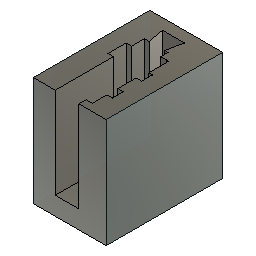
Endstop8 v4 (Autodesk Fusion 360 design; units mm, degrees)
Autodesk Fusion 360 part; units mm, degrees
note: some values were not read from the file. Chosen so that the rebuilt part matches the saved one: which face or edge a step refers to. Set by a fixed rule: which sketch regions a step uses.
(part 1 of 2)
sketch "Skizze1" plane through (0, 0, 0) normal (0, 0, 1) x (1, 0, 0)
  line L0 (0, 0) -> (20, 0)
  line L1 (20, 0) -> (20, -32)
  line L2 (20, -32) -> (0, -32)
  line L3 (0, -32) -> (0, 0)
  dimension "d1" = 20
  dimension "d2" = 32
  constraint horizontal L0
  constraint vertical L1
  constraint horizontal L2
  constraint vertical L3
  constraint coincident L0.start L3.end
  measures "d1" distance of L0.start L0.end
  measures "d2" distance of L0.start L2.end
extrude "Extrusion1" add sketch "Skizze1" along normal blind 25
sketch "Skizze2" plane through (0, 0, 25) normal (0, 0, 1) x (-1, 0, 0)
  line L0 (0, 32) -> (-20, 32)
  line L1 (-20, 32) -> (-20, 0)
  line L2 (-20, 0) -> (0, 0)
  line L3 (0, 0) -> (0, 32)
  line L4 (-12.516, 32) -> (-4.516, 32)
  line L5 (-4.516, 32) -> (-4.516, 10)
  line L6 (-4.516, 10) -> (-12.516, 10)
  line L7 (-12.516, 10) -> (-12.516, 32)
  dimension "d5" = 8
  dimension "d6" = 22
  constraint horizontal L4
  constraint vertical L5
  constraint horizontal L6
  constraint vertical L7
  constraint coincident L0 L4.start
  measures "d5" distance of L4.start L4.end
  measures "d6" distance of L4.start L6.end
extrude "Extrusion2" cut sketch "Skizze2" against normal blind 100 contours L0 L4 L5 L6 L7
sketch "Skizze3" plane through (0, 0, 25) normal (0, 0, 1) x (-1, 0, 0)
  line L0 (-12.516, 10) -> (-12.516, 32)
  line L1 (-12.516, 32) -> (-20, 32)
  line L2 (-20, 32) -> (-20, 0)
  line L3 (-20, 0) -> (0, 0)
  line L4 (0, 0) -> (0, 32)
  line L5 (0, 32) -> (-4.516, 32)
  line L6 (-4.516, 32) -> (-4.516, 10)
  line L7 (-4.516, 10) -> (-12.516, 10)
  line L8 (-12.516, 25.5233) -> (-14.516, 25.5233)
  line L9 (-14.516, 25.5233) -> (-14.516, 23.5233)
  line L10 (-14.516, 23.5233) -> (-12.516, 23.5233)
  line L11 (-12.516, 23.5233) -> (-12.516, 25.5233)
  dimension "d9" = 2
  dimension "d10" = 2
  constraint horizontal L8
  constraint vertical L9
  constraint horizontal L10
  constraint vertical L11
  constraint coincident L0 L8.start
  measures "d9" distance of L8.start L8.end
  measures "d10" distance of L8.start L10.end
extrude "Extrusion3" cut sketch "Skizze3" against normal blind 100 contours L0 L8 L9 L10 L11
sketch "Skizze4" plane through (0, 0, 25) normal (0, 0, 1) x (-1, 0, 0)
  line L0 (-14.516, 25.5233) -> (-12.516, 25.5233)
  line L1 (-12.516, 25.5233) -> (-12.516, 32)
  line L2 (-12.516, 32) -> (-20, 32)
  line L3 (-20, 32) -> (-20, 0)
  line L4 (-20, 0) -> (0, 0)
  line L5 (0, 0) -> (0, 32)
  line L6 (0, 32) -> (-4.516, 32)
  line L7 (-4.516, 32) -> (-4.516, 10)
  line L8 (-4.516, 10) -> (-12.516, 10)
  line L9 (-12.516, 10) -> (-12.516, 23.5233)
  line L10 (-12.516, 23.5233) -> (-14.516, 23.5233)
  line L11 (-14.516, 23.5233) -> (-14.516, 25.5233)
  line L12 (-12.516, 17.5114) -> (-14.516, 17.5114)
  line L13 (-14.516, 17.5114) -> (-14.516, 15.5114)
  line L14 (-14.516, 15.5114) -> (-12.516, 15.5114)
  line L15 (-12.516, 15.5114) -> (-12.516, 17.5114)
  dimension "d13" = 2
  dimension "d14" = 2
  constraint horizontal L12
  constraint vertical L13
  constraint horizontal L14
  constraint vertical L15
  constraint coincident L9 L12.start
  measures "d13" distance of L12.start L12.end
  measures "d14" distance of L12.start L14.end
extrude "Extrusion4" cut sketch "Skizze4" against normal blind 100 contours L9 L12 L13 L14 L15
sketch "Skizze5" plane through (0, 0, 25) normal (0, 0, 1) x (-1, 0, 0)
  line L0 (-12.516, 15.5114) -> (-14.516, 15.5114)
  line L1 (-14.516, 15.5114) -> (-14.516, 17.5114)
  line L2 (-14.516, 17.5114) -> (-12.516, 17.5114)
  line L3 (-12.516, 17.5114) -> (-12.516, 23.5233)
  line L4 (-12.516, 23.5233) -> (-14.516, 23.5233)
  line L5 (-14.516, 23.5233) -> (-14.516, 25.5233)
  line L6 (-14.516, 25.5233) -> (-12.516, 25.5233)
  line L7 (-12.516, 25.5233) -> (-12.516, 32)
  line L8 (-12.516, 32) -> (-20, 32)
  line L9 (-20, 32) -> (-20, 0)
  line L10 (-20, 0) -> (0, 0)
  line L11 (0, 0) -> (0, 32)
  line L12 (0, 32) -> (-4.516, 32)
  line L13 (-4.516, 32) -> (-4.516, 10)
  line L14 (-4.516, 10) -> (-12.516, 10)
  line L15 (-12.516, 10) -> (-12.516, 15.5114)
  line L16 (-12.516, 30.0118) -> (-14.216, 30.0118)
  line L17 (-14.216, 30.0118) -> (-14.216, 10.0118)
  line L18 (-14.216, 10.0118) -> (-12.516, 10.0118)
  line L19 (-12.516, 10.0118) -> (-12.516, 30.0118)
  dimension "d17" = 1.7
  dimension "d18" = 20
  constraint horizontal L16
  constraint vertical L17
  constraint horizontal L18
  constraint vertical L19
  constraint coincident L7 L16.start
  measures "d17" distance of L16.start L16.end
  measures "d18" distance of L16.start L18.end
extrude "Extrusion5" cut sketch "Skizze5" against normal blind 100 contours L0 L15 L17 L18 L19 | L2 L3 L4 L17 L19 | L6 L7 L16 L17 L19
sketch "Skizze6" plane through (0, 0, 25) normal (0, 0, 1) x (-1, 0, 0)
  line L0 (-12.516, 10.0118) -> (-14.216, 10.0118)
  line L1 (-14.216, 10.0118) -> (-14.216, 15.5114)
  line L2 (-14.216, 15.5114) -> (-14.516, 15.5114)
  line L3 (-14.516, 15.5114) -> (-14.516, 17.5114)
  line L4 (-14.516, 17.5114) -> (-14.216, 17.5114)
  line L5 (-14.216, 17.5114) -> (-14.216, 23.5233)
  line L6 (-14.216, 23.5233) -> (-14.516, 23.5233)
  line L7 (-14.516, 23.5233) -> (-14.516, 25.5233)
  line L8 (-14.516, 25.5233) -> (-14.216, 25.5233)
  line L9 (-14.216, 25.5233) -> (-14.216, 30.0118)
  line L10 (-14.216, 30.0118) -> (-12.516, 30.0118)
  line L11 (-12.516, 30.0118) -> (-12.516, 32)
  line L12 (-12.516, 32) -> (-20, 32)
  line L13 (-20, 32) -> (-20, 0)
  line L14 (-20, 0) -> (0, 0)
  line L15 (0, 0) -> (0, 32)
  line L16 (0, 32) -> (-4.516, 32)
  line L17 (-4.516, 32) -> (-4.516, 10)
  line L18 (-4.516, 10) -> (-12.516, 10)
  line L19 (-12.516, 10) -> (-12.516, 10.0118)
  line L20 (-14.516, 23.5233) -> (-15.716, 23.5233)
  line L21 (-15.716, 23.5233) -> (-15.716, 25.5)
  line L22 (-15.716, 25.5) -> (-14.516, 25.5)
  line L23 (-14.516, 25.5) -> (-14.516, 23.5233)
  dimension "d21" = 1.2
  constraint horizontal L20
  constraint vertical L21
  constraint horizontal L22
  constraint vertical L23
  constraint coincident L6.end L7.start
  measures "d21" distance of L6.end L20.end
extrude "Extrusion6" cut sketch "Skizze6" against normal blind 100 contours L7 L20 L21 L22 L23
sketch "Skizze7" plane through (0, 0, 25) normal (0, 0, 1) x (-1, 0, 0)
  line L0 (-14.216, 23.5233) -> (-15.716, 23.5233)
  line L1 (-15.716, 23.5233) -> (-15.716, 25.5)
  line L2 (-15.716, 25.5) -> (-14.516, 25.5)
  line L3 (-14.516, 25.5) -> (-14.516, 25.5233)
  line L4 (-14.516, 25.5233) -> (-14.216, 25.5233)
  line L5 (-14.216, 25.5233) -> (-14.216, 30.0118)
  line L6 (-14.216, 30.0118) -> (-12.516, 30.0118)
  line L7 (-12.516, 30.0118) -> (-12.516, 32)
  line L8 (-12.516, 32) -> (-20, 32)
  line L9 (-20, 32) -> (-20, 0)
  line L10 (-20, 0) -> (0, 0)
  line L11 (0, 0) -> (0, 32)
  line L12 (0, 32) -> (-4.516, 32)
  line L13 (-4.516, 32) -> (-4.516, 10)
  line L14 (-4.516, 10) -> (-12.516, 10)
  line L15 (-12.516, 10) -> (-12.516, 10.0118)
  line L16 (-12.516, 10.0118) -> (-14.216, 10.0118)
  line L17 (-14.216, 10.0118) -> (-14.216, 15.5114)
  line L18 (-14.216, 15.5114) -> (-14.516, 15.5114)
  line L19 (-14.516, 15.5114) -> (-14.516, 17.5114)
  line L20 (-14.516, 17.5114) -> (-14.216, 17.5114)
  line L21 (-14.216, 17.5114) -> (-14.216, 23.5233)
  line L22 (-14.516, 17.5114) -> (-15.716, 17.5114)
  line L23 (-15.716, 17.5114) -> (-15.716, 15.5)
  line L24 (-15.716, 15.5) -> (-14.516, 15.5)
  line L25 (-14.516, 15.5) -> (-14.516, 17.5114)
  dimension "d24" = 1.2
  constraint horizontal L22
  constraint vertical L23
  constraint horizontal L24
  constraint vertical L25
  constraint coincident L19.end L20.start
  measures "d24" distance of L19.end L22.end
extrude "Extrusion7" cut sketch "Skizze7" against normal blind 100 contours L19 L22 L23 L24 L25
sketch "Skizze8" plane through (0, 0, 25) normal (0, 0, 1) x (-1, 0, 0)
  line L0 (-14.516, 15.5114) -> (-14.516, 15.5)
  line L1 (-14.516, 15.5) -> (-15.716, 15.5)
  line L2 (-15.716, 15.5) -> (-15.716, 17.5114)
  line L3 (-15.716, 17.5114) -> (-14.216, 17.5114)
  line L4 (-14.216, 17.5114) -> (-14.216, 23.5233)
  line L5 (-14.216, 23.5233) -> (-15.716, 23.5233)
  line L6 (-15.716, 23.5233) -> (-15.716, 25.5)
  line L7 (-15.716, 25.5) -> (-14.516, 25.5)
  line L8 (-14.516, 25.5) -> (-14.516, 25.5233)
  line L9 (-14.516, 25.5233) -> (-14.216, 25.5233)
  line L10 (-14.216, 25.5233) -> (-14.216, 30.0118)
  line L11 (-14.216, 30.0118) -> (-12.516, 30.0118)
  line L12 (-12.516, 30.0118) -> (-12.516, 32)
  line L13 (-12.516, 32) -> (-20, 32)
  line L14 (-20, 32) -> (-20, 0)
  line L15 (-20, 0) -> (0, 0)
  line L16 (0, 0) -> (0, 32)
  line L17 (0, 32) -> (-4.516, 32)
  line L18 (-4.516, 32) -> (-4.516, 10)
  line L19 (-4.516, 10) -> (-12.516, 10)
  line L20 (-12.516, 10) -> (-12.516, 10.0118)
  line L21 (-12.516, 10.0118) -> (-14.216, 10.0118)
  line L22 (-14.216, 10.0118) -> (-14.216, 15.5114)
  line L23 (-14.216, 15.5114) -> (-14.516, 15.5114)
  line L24 (-12.516, 10) -> (-4.516, 10)
  line L25 (-4.516, 10) -> (-4.516, 8)
  line L26 (-4.516, 8) -> (-12.516, 8)
  line L27 (-12.516, 8) -> (-12.516, 10)
  dimension "d27" = 8
  dimension "d28" = 2
  constraint horizontal L24
  constraint vertical L25
  constraint horizontal L26
  constraint vertical L27
  constraint coincident L19.end L20.start
  measures "d27" distance of L19.end L18.end
  measures "d28" distance of L19.end L26.end
extrude "Extrusion8" cut sketch "Skizze8" against normal blind 100 contours L19 L24 L25 L26 L27
hole "Bohrung1" at (8.516, -8, 25) direction (0, 0, -1) diameter 8 depth 1000 tip angle 180
sketch "Skizze12" plane through (0, 0, 25) normal (0, 0, 1) x (-1, 0, 0)
  arc A0 (-12.516, 8) -> (-4.516, 8) centre (-8.516, 8) ccw
  line L0 (-12.516, 8) -> (-12.516, 10.0118)
  line L1 (-12.516, 10.0118) -> (-14.216, 10.0118)
  line L2 (-14.216, 10.0118) -> (-14.216, 15.5114)
  line L3 (-14.216, 15.5114) -> (-14.516, 15.5114)
  line L4 (-14.516, 15.5114) -> (-14.516, 15.5)
  line L5 (-14.516, 15.5) -> (-15.716, 15.5)
  line L6 (-15.716, 15.5) -> (-15.716, 17.5114)
  line L7 (-15.716, 17.5114) -> (-14.216, 17.5114)
  line L8 (-14.216, 17.5114) -> (-14.216, 23.5233)
  line L9 (-14.216, 23.5233) -> (-15.716, 23.5233)
  line L10 (-15.716, 23.5233) -> (-15.716, 25.5)
  line L11 (-15.716, 25.5) -> (-14.516, 25.5)
  line L12 (-14.516, 25.5) -> (-14.516, 25.5233)
  line L13 (-14.516, 25.5233) -> (-14.216, 25.5233)
  line L14 (-14.216, 25.5233) -> (-14.216, 30.0118)
  line L15 (-14.216, 30.0118) -> (-12.516, 30.0118)
  line L16 (-12.516, 30.0118) -> (-12.516, 32)
  line L17 (-12.516, 32) -> (-20, 32)
  line L18 (-20, 32) -> (-20, 0)
  line L19 (-20, 0) -> (0, 0)
  line L20 (0, 0) -> (0, 32)
  line L21 (0, 32) -> (-4.516, 32)
  line L22 (-4.516, 32) -> (-4.516, 8)
  line L23 (-12.516, 10.0118) -> (-14.216, 10.0118)
  line L24 (-14.216, 10.0118) -> (-14.216, 9.5118)
  line L25 (-14.216, 9.5118) -> (-12.516, 9.5118)
  line L26 (-12.516, 9.5118) -> (-12.516, 10.0118)
  line L27 (-14.216, 14.9916) -> (-15.716, 14.9916)
  line L28 (-15.716, 14.9916) -> (-15.716, 17.9916)
  line L29 (-15.716, 17.9916) -> (-14.216, 17.9916)
  line L30 (-14.216, 17.9916) -> (-14.216, 14.9916)
  line L31 (-14.216, 23.0062) -> (-15.716, 23.0062)
  line L32 (-15.716, 23.0062) -> (-15.716, 26.0062)
  line L33 (-15.716, 26.0062) -> (-14.216, 26.0062)
  line L34 (-14.216, 26.0062) -> (-14.216, 23.0062)
  dimension "d47" = 1.7
  dimension "d48" = 0.5
  dimension "d49" = 1.5
  dimension "d50" = 3
  dimension "d51" = 1.5
  dimension "d52" = 3
  constraint horizontal L23
  constraint vertical L24
  constraint horizontal L25
  constraint vertical L26
  constraint coincident L0.end L1.start
  constraint horizontal L27
  constraint vertical L28
  constraint horizontal L29
  constraint vertical L30
  constraint coincident L2 L27.start
  constraint horizontal L31
  constraint vertical L32
  constraint horizontal L33
  constraint vertical L34
  constraint coincident L8 L31.start
  measures "d47" distance of L0.end L1.end
  measures "d48" distance of L0.end L25.end
  measures "d49" distance of L27.start L27.end
  measures "d50" distance of L27.start L29.end
  measures "d51" distance of L31.start L31.end
  measures "d52" distance of L31.start L33.end
extrude "Extrusion12" cut sketch "Skizze12" against normal blind 100 contours L0 L1 L23 L24 L25 L26 | L2 L3 L4 L5 L27 L28 L30 | L7 L8 L28 L29 L30 | L8 L9 L31 L32 L34 | L11 L12 L13 L14 L32 L33 L34
sketch "Skizze13" plane through (0, 0, 25) normal (0, 0, 1) x (-1, 0, 0)
  line L0 (-15.716, 14.9916) -> (-15.716, 17.9916)
  line L1 (-15.716, 17.9916) -> (-14.216, 17.9916)
  line L2 (-14.216, 17.9916) -> (-14.216, 23.0062)
  line L3 (-14.216, 23.0062) -> (-15.716, 23.0062)
  line L4 (-15.716, 23.0062) -> (-15.716, 26.0062)
  line L5 (-15.716, 26.0062) -> (-14.216, 26.0062)
  line L6 (-14.216, 26.0062) -> (-14.216, 30.0118)
  line L7 (-14.216, 30.0118) -> (-12.516, 30.0118)
  line L8 (-12.516, 30.0118) -> (-12.516, 32)
  line L9 (-12.516, 32) -> (-20, 32)
  line L10 (-20, 32) -> (-20, 0)
  line L11 (-20, 0) -> (0, 0)
  line L12 (0, 0) -> (0, 32)
  line L13 (0, 32) -> (-4.516, 32)
  line L14 (-4.516, 32) -> (-4.516, 8)
  arc A0 (-12.516, 8) -> (-4.516, 8) centre (-8.516, 8) ccw
  line L15 (-12.516, 8) -> (-12.516, 9.5118)
  line L16 (-12.516, 9.5118) -> (-14.216, 9.5118)
  line L17 (-14.216, 9.5118) -> (-14.216, 14.9916)
  line L18 (-14.216, 14.9916) -> (-15.716, 14.9916)
  line L19 (-12.516, 8) -> (-10, 8)
  line L20 (-10, 8) -> (-10, 4.2855)
  constraint coincident A0.start L15.start
  constraint perpendicular L15 L19
  constraint coincident A0 L20.end
  constraint perpendicular L19 L20
extrude "Extrusion13" add sketch "Skizze13" against normal blind 25 contours A0 L19 L20
sketch "Skizze14" plane through (0, 0, 25) normal (0, 0, 1) x (-1, 0, 0)
  line L0 (-15.716, 14.9916) -> (-15.716, 17.9916)
  line L1 (-15.716, 17.9916) -> (-14.216, 17.9916)
  line L2 (-14.216, 17.9916) -> (-14.216, 23.0062)
  line L3 (-14.216, 23.0062) -> (-15.716, 23.0062)
  line L4 (-15.716, 23.0062) -> (-15.716, 26.0062)
  line L5 (-15.716, 26.0062) -> (-14.216, 26.0062)
  line L6 (-14.216, 26.0062) -> (-14.216, 30.0118)
  line L7 (-14.216, 30.0118) -> (-12.516, 30.0118)
  line L8 (-12.516, 30.0118) -> (-12.516, 32)
  line L9 (-12.516, 32) -> (-20, 32)
  line L10 (-20, 32) -> (-20, 0)
  line L11 (-20, 0) -> (0, 0)
  line L12 (0, 0) -> (0, 32)
  line L13 (0, 32) -> (-4.516, 32)
  line L14 (-4.516, 32) -> (-4.516, 8)
  arc A0 (-10, 4.2855) -> (-4.516, 8) centre (-8.516, 8) ccw
  line L15 (-10, 4.2855) -> (-10, 8)
  line L16 (-10, 8) -> (-12.516, 8)
  line L17 (-12.516, 8) -> (-12.516, 9.5118)
  line L18 (-12.516, 9.5118) -> (-14.216, 9.5118)
  line L19 (-14.216, 9.5118) -> (-14.216, 14.9916)
  line L20 (-14.216, 14.9916) -> (-15.716, 14.9916)
  line L21 (-7.0738, 4.269) -> (-7.0738, 8)
  line L22 (-7.0738, 8) -> (-4.516, 8)
  constraint coincident A0 L21.start
  constraint parallel L12 L21
  constraint coincident L14.end A0.end
extrude "Extrusion14" add sketch "Skizze14" against normal blind 25 contours A0 L21 L22
sketch "Skizze15" plane through (0, 0, 25) normal (0, 0, 1) x (-1, 0, 0)
  line L0 (-15.716, 14.9916) -> (-15.716, 17.9916)
  line L1 (-15.716, 17.9916) -> (-14.216, 17.9916)
  line L2 (-14.216, 17.9916) -> (-14.216, 23.0062)
  line L3 (-14.216, 23.0062) -> (-15.716, 23.0062)
  line L4 (-15.716, 23.0062) -> (-15.716, 26.0062)
  line L5 (-15.716, 26.0062) -> (-14.216, 26.0062)
  line L6 (-14.216, 26.0062) -> (-14.216, 30.0118)
  line L7 (-14.216, 30.0118) -> (-12.516, 30.0118)
  line L8 (-12.516, 30.0118) -> (-12.516, 32)
  line L9 (-12.516, 32) -> (-20, 32)
  line L10 (-20, 32) -> (-20, 0)
  line L11 (-20, 0) -> (0, 0)
  line L12 (0, 0) -> (0, 32)
  line L13 (0, 32) -> (-4.516, 32)
  line L14 (-4.516, 32) -> (-4.516, 8)
  line L15 (-4.516, 8) -> (-7.0738, 8)
  line L16 (-7.0738, 8) -> (-7.0738, 4.269)
  arc A0 (-10, 4.2855) -> (-7.0738, 4.269) centre (-8.516, 8) ccw
  line L17 (-10, 4.2855) -> (-10, 8)
  line L18 (-10, 8) -> (-12.516, 8)
  line L19 (-12.516, 8) -> (-12.516, 9.5118)
  line L20 (-12.516, 9.5118) -> (-14.216, 9.5118)
  line L21 (-14.216, 9.5118) -> (-14.216, 14.9916)
  line L22 (-14.216, 14.9916) -> (-15.716, 14.9916)
  line L23 (-7.0738, 8) -> (-6.6738, 8)
  line L24 (-6.6738, 8) -> (-6.6738, 4.0061)
  line L25 (-6.6738, 4.0061) -> (-7.0738, 4.0061)
  line L26 (-7.0738, 4.0061) -> (-7.0738, 8)
  line L27 (-10, 8) -> (-10.4, 8)
  line L28 (-10.4, 8) -> (-10.4, 4.0061)
  line L29 (-10.4, 4.0061) -> (-10, 4.0061)
  line L30 (-10, 4.0061) -> (-10, 8)
  line L31 (-6.6738, 4.0061) -> (-10.4, 4.0061)
  line L32 (-10.4, 4.0061) -> (-10.4, 4.5457)
  line L33 (-10.4, 4.5457) -> (-6.6738, 4.5457)
  line L34 (-6.6738, 4.5457) -> (-6.6738, 4.0061)
  dimension "d59" = 0.4
  dimension "d60" = 0.4
  constraint horizontal L23
  constraint vertical L24
  constraint horizontal L25
  constraint vertical L26
  constraint coincident L15.end L16.start
  constraint horizontal L27
  constraint vertical L28
  constraint horizontal L29
  constraint vertical L30
  constraint coincident L17.end L18.start
  constraint horizontal L31
  constraint vertical L32
  constraint horizontal L33
  constraint vertical L34
  constraint coincident L28 L32.end
  measures "d59" distance of L15.end L23.end
  measures "d60" distance of L17.end L27.end
extrude "Extrusion15" cut sketch "Skizze15" against normal blind 30 contours L17 L18 L27 L28 L30 L33 | L17 L28 L29 L30 L31 L32 L33 | A0 L30 L31 | L16 L24 L25 L26 L31 L33 L34 | L15 L16 L23 L24 L26 L33 | A0 L26 L31
sketch "Skizze16" plane through (0, 0, 25) normal (0, 0, 1) x (-1, 0, 0)
  line L0 (-6.6738, 8) -> (-6.6738, 4.0061)
  line L1 (-6.6738, 4.0061) -> (-8.2952, 4.0061)
  arc A0 (-8.7369, 4.0061) -> (-8.2952, 4.0061) centre (-8.516, 8) ccw
  line L2 (-8.7369, 4.0061) -> (-10.4, 4.0061)
  line L3 (-10.4, 4.0061) -> (-10.4, 8)
  line L4 (-10.4, 8) -> (-12.516, 8)
  line L5 (-12.516, 8) -> (-12.516, 9.5118)
  line L6 (-12.516, 9.5118) -> (-14.216, 9.5118)
  line L7 (-14.216, 9.5118) -> (-14.216, 14.9916)
  line L8 (-14.216, 14.9916) -> (-15.716, 14.9916)
  line L9 (-15.716, 14.9916) -> (-15.716, 17.9916)
  line L10 (-15.716, 17.9916) -> (-14.216, 17.9916)
  line L11 (-14.216, 17.9916) -> (-14.216, 23.0062)
  line L12 (-14.216, 23.0062) -> (-15.716, 23.0062)
  line L13 (-15.716, 23.0062) -> (-15.716, 26.0062)
  line L14 (-15.716, 26.0062) -> (-14.216, 26.0062)
  line L15 (-14.216, 26.0062) -> (-14.216, 30.0118)
  line L16 (-14.216, 30.0118) -> (-12.516, 30.0118)
  line L17 (-12.516, 30.0118) -> (-12.516, 32)
  line L18 (-12.516, 32) -> (-20, 32)
  line L19 (-20, 32) -> (-20, 0)
  line L20 (-20, 0) -> (0, 0)
  line L21 (0, 0) -> (0, 32)
  line L22 (0, 32) -> (-4.516, 32)
  line L23 (-4.516, 32) -> (-4.516, 8)
  line L24 (-4.516, 8) -> (-6.6738, 8)
  line L25 (-4.516, 32) -> (-6.016, 32)
  line L26 (-6.016, 32) -> (-6.016, 8)
  line L27 (-6.016, 8) -> (-4.516, 8)
  line L28 (-4.516, 8) -> (-4.516, 32)
  dimension "d63" = 1.5
  constraint horizontal L25
  constraint vertical L26
  constraint horizontal L27
  constraint vertical L28
  constraint coincident L22.end L23.start
  measures "d63" distance of L22.end L25.end
extrude "Extrusion16" add sketch "Skizze16" against normal blind 25 contours L23 L24 L25 L26 L27 L28
sketch "Skizze17" plane through (0, 0, 25) normal (0, 0, 1) x (-1, 0, 0)
  line L0 (-6.6738, 8) -> (-6.6738, 4.0061)
  line L1 (-6.6738, 4.0061) -> (-8.2952, 4.0061)
  arc A0 (-8.7369, 4.0061) -> (-8.2952, 4.0061) centre (-8.516, 8) ccw
  line L2 (-8.7369, 4.0061) -> (-10.4, 4.0061)
  line L3 (-10.4, 4.0061) -> (-10.4, 8)
  line L4 (-10.4, 8) -> (-12.516, 8)
  line L5 (-12.516, 8) -> (-12.516, 9.5118)
  line L6 (-12.516, 9.5118) -> (-14.216, 9.5118)
  line L7 (-14.216, 9.5118) -> (-14.216, 14.9916)
  line L8 (-14.216, 14.9916) -> (-15.716, 14.9916)
  line L9 (-15.716, 14.9916) -> (-15.716, 17.9916)
  line L10 (-15.716, 17.9916) -> (-14.216, 17.9916)
  line L11 (-14.216, 17.9916) -> (-14.216, 23.0062)
  line L12 (-14.216, 23.0062) -> (-15.716, 23.0062)
  line L13 (-15.716, 23.0062) -> (-15.716, 26.0062)
  line L14 (-15.716, 26.0062) -> (-14.216, 26.0062)
  line L15 (-14.216, 26.0062) -> (-14.216, 30.0118)
  line L16 (-14.216, 30.0118) -> (-12.516, 30.0118)
  line L17 (-12.516, 30.0118) -> (-12.516, 32)
  line L18 (-12.516, 32) -> (-20, 32)
  line L19 (-20, 32) -> (-20, 0)
  line L20 (-20, 0) -> (0, 0)
  line L21 (0, 0) -> (0, 32)
  line L22 (0, 32) -> (-6.016, 32)
  line L23 (-6.016, 32) -> (-6.016, 8)
  line L24 (-6.016, 8) -> (-6.6738, 8)
  line L25 (-14.216, 14.9916) -> (-14.716, 14.9916)
  line L26 (-14.716, 14.9916) -> (-14.716, 9.513)
  line L27 (-14.716, 9.513) -> (-14.216, 9.513)
  line L28 (-14.216, 9.513) -> (-14.216, 14.9916)
  dimension "d66" = 0.5
  constraint horizontal L25
  constraint vertical L26
  constraint horizontal L27
  constraint vertical L28
  constraint coincident L7.end L8.start
  measures "d66" distance of L7.end L25.end
extrude "Extrusion17" cut sketch "Skizze17" against normal blind 25 contours L7 L8 L25 L26 L27 L28
sketch "Skizze18" plane through (0, 0, 25) normal (0, 0, 1) x (-1, 0, 0)
  line L0 (-14.216, 9.513) -> (-14.716, 9.513)
  line L1 (-14.716, 9.513) -> (-14.716, 14.9916)
  line L2 (-14.716, 14.9916) -> (-15.716, 14.9916)
  line L3 (-15.716, 14.9916) -> (-15.716, 17.9916)
  line L4 (-15.716, 17.9916) -> (-14.216, 17.9916)
  line L5 (-14.216, 17.9916) -> (-14.216, 23.0062)
  line L6 (-14.216, 23.0062) -> (-15.716, 23.0062)
  line L7 (-15.716, 23.0062) -> (-15.716, 26.0062)
  line L8 (-15.716, 26.0062) -> (-14.216, 26.0062)
  line L9 (-14.216, 26.0062) -> (-14.216, 30.0118)
  line L10 (-14.216, 30.0118) -> (-12.516, 30.0118)
  line L11 (-12.516, 30.0118) -> (-12.516, 32)
  line L12 (-12.516, 32) -> (-20, 32)
  line L13 (-20, 32) -> (-20, 0)
  line L14 (-20, 0) -> (0, 0)
  line L15 (0, 0) -> (0, 32)
  line L16 (0, 32) -> (-6.016, 32)
  line L17 (-6.016, 32) -> (-6.016, 8)
  line L18 (-6.016, 8) -> (-6.6738, 8)
  line L19 (-6.6738, 8) -> (-6.6738, 4.0061)
  line L20 (-6.6738, 4.0061) -> (-8.2952, 4.0061)
  arc A0 (-8.7369, 4.0061) -> (-8.2952, 4.0061) centre (-8.516, 8) ccw
  line L21 (-8.7369, 4.0061) -> (-10.4, 4.0061)
  line L22 (-10.4, 4.0061) -> (-10.4, 8)
  line L23 (-10.4, 8) -> (-12.516, 8)
  line L24 (-12.516, 8) -> (-12.516, 9.5118)
  line L25 (-12.516, 9.5118) -> (-14.216, 9.5118)
  line L26 (-14.216, 9.5118) -> (-14.216, 9.513)
  line L27 (-10.4, 8) -> (-11.4, 8)
  line L28 (-11.4, 8) -> (-11.4, 4.0168)
  line L29 (-11.4, 4.0168) -> (-10.4, 4.0168)
  line L30 (-10.4, 4.0168) -> (-10.4, 8)
  line L31 (-10.4, 8) -> (-11.6, 8)
  line L32 (-11.6, 8) -> (-11.6, 4.008)
  line L33 (-11.6, 4.008) -> (-10.4, 4.008)
  line L34 (-10.4, 4.008) -> (-10.4, 8)
  point P0 (-10.4, 4.0061)
  point P1 (-10.4, 8)
  point P2 (-10.4, 4.0061)
  dimension "d69" = 1
  dimension "d70" = 1.2
  constraint horizontal L27
  constraint vertical L28
  constraint horizontal L29
  constraint vertical L30
  constraint horizontal L31
  constraint vertical L32
  constraint horizontal L33
  constraint vertical L34
  measures "d69" distance of P1 L27.end
  measures "d70" distance of P1 L31.end
extrude "Extrusion18" cut sketch "Skizze18" against normal blind 30 contours L22 L23 L28 L29 L31 L32 L33 L34 | L22 L23 L27 L28 L29 L30 L31 L34
sketch "Skizze19" plane through (0, 0, 25) normal (0, 0, 1) x (-1, 0, 0)
  line L0 (-10.4, 4.008) -> (-11.6, 4.008)
  line L1 (-11.6, 4.008) -> (-11.6, 8)
  line L2 (-11.6, 8) -> (-12.516, 8)
  line L3 (-12.516, 8) -> (-12.516, 9.5118)
  line L4 (-12.516, 9.5118) -> (-14.216, 9.5118)
  line L5 (-14.216, 9.5118) -> (-14.216, 9.513)
  line L6 (-14.216, 9.513) -> (-14.716, 9.513)
  line L7 (-14.716, 9.513) -> (-14.716, 14.9916)
  line L8 (-14.716, 14.9916) -> (-15.716, 14.9916)
  line L9 (-15.716, 14.9916) -> (-15.716, 17.9916)
  line L10 (-15.716, 17.9916) -> (-14.216, 17.9916)
  line L11 (-14.216, 17.9916) -> (-14.216, 23.0062)
  line L12 (-14.216, 23.0062) -> (-15.716, 23.0062)
  line L13 (-15.716, 23.0062) -> (-15.716, 26.0062)
  line L14 (-15.716, 26.0062) -> (-14.216, 26.0062)
  line L15 (-14.216, 26.0062) -> (-14.216, 30.0118)
  line L16 (-14.216, 30.0118) -> (-12.516, 30.0118)
  line L17 (-12.516, 30.0118) -> (-12.516, 32)
  line L18 (-12.516, 32) -> (-20, 32)
  line L19 (-20, 32) -> (-20, 0)
  line L20 (-20, 0) -> (0, 0)
  line L21 (0, 0) -> (0, 32)
  line L22 (0, 32) -> (-6.016, 32)
  line L23 (-6.016, 32) -> (-6.016, 8)
  line L24 (-6.016, 8) -> (-6.6738, 8)
  line L25 (-6.6738, 8) -> (-6.6738, 4.0061)
  line L26 (-6.6738, 4.0061) -> (-8.2952, 4.0061)
  arc A0 (-8.7369, 4.0061) -> (-8.2952, 4.0061) centre (-8.516, 8) ccw
  line L27 (-8.7369, 4.0061) -> (-10.4, 4.0061)
  line L28 (-10.4, 4.0061) -> (-10.4, 4.008)
  line L29 (-6.016, 8) -> (-12.5254, 8)
  line L30 (-12.5254, 8) -> (-12.5254, 7.5)
  line L31 (-12.5254, 7.5) -> (-6.016, 7.5)
  line L32 (-6.016, 7.5) -> (-6.016, 8)
  dimension "d73" = 0.5
  constraint horizontal L29
  constraint vertical L30
  constraint horizontal L31
  constraint vertical L32
  constraint coincident L23.end L24.start
  measures "d73" distance of L23.end L31.end
extrude "Extrusion19" cut sketch "Skizze19" against normal blind 30 contours L1 L2 L29 L30 L31 | L24 L25 L29 L31 L32
sketch "Skizze20" plane through (0, 0, 25) normal (0, 0, 1) x (-1, 0, 0)
  line L0 (-6.016, 7.5) -> (-6.6738, 7.5)
  line L1 (-6.6738, 7.5) -> (-6.6738, 4.0061)
  line L2 (-6.6738, 4.0061) -> (-8.2952, 4.0061)
  arc A0 (-8.7369, 4.0061) -> (-8.2952, 4.0061) centre (-8.516, 8) ccw
  line L3 (-8.7369, 4.0061) -> (-10.4, 4.0061)
  line L4 (-10.4, 4.0061) -> (-10.4, 4.008)
  line L5 (-10.4, 4.008) -> (-11.6, 4.008)
  line L6 (-11.6, 4.008) -> (-11.6, 7.5)
  line L7 (-11.6, 7.5) -> (-12.5254, 7.5)
  line L8 (-12.5254, 7.5) -> (-12.5254, 8)
  line L9 (-12.5254, 8) -> (-12.516, 8)
  line L10 (-12.516, 8) -> (-12.516, 9.5118)
  line L11 (-12.516, 9.5118) -> (-14.216, 9.5118)
  line L12 (-14.216, 9.5118) -> (-14.216, 9.513)
  line L13 (-14.216, 9.513) -> (-14.716, 9.513)
  line L14 (-14.716, 9.513) -> (-14.716, 14.9916)
  line L15 (-14.716, 14.9916) -> (-15.716, 14.9916)
  line L16 (-15.716, 14.9916) -> (-15.716, 17.9916)
  line L17 (-15.716, 17.9916) -> (-14.216, 17.9916)
  line L18 (-14.216, 17.9916) -> (-14.216, 23.0062)
  line L19 (-14.216, 23.0062) -> (-15.716, 23.0062)
  line L20 (-15.716, 23.0062) -> (-15.716, 26.0062)
  line L21 (-15.716, 26.0062) -> (-14.216, 26.0062)
  line L22 (-14.216, 26.0062) -> (-14.216, 30.0118)
  line L23 (-14.216, 30.0118) -> (-12.516, 30.0118)
  line L24 (-12.516, 30.0118) -> (-12.516, 32)
  line L25 (-12.516, 32) -> (-20, 32)
  line L26 (-20, 32) -> (-20, 0)
  line L27 (-20, 0) -> (0, 0)
  line L28 (0, 0) -> (0, 32)
  line L29 (0, 32) -> (-6.016, 32)
  line L30 (-6.016, 32) -> (-6.016, 7.5)
  line L31 (-6.016, 15.0187) -> (-4.516, 15.0187)
  line L32 (-4.516, 15.0187) -> (-4.516, 12.0187)
  line L33 (-4.516, 12.0187) -> (-6.016, 12.0187)
  line L34 (-6.016, 12.0187) -> (-6.016, 15.0187)
  dimension "d76" = 1.5
  dimension "d77" = 3
  constraint horizontal L31
  constraint vertical L32
  constraint horizontal L33
  constraint vertical L34
  constraint coincident L30 L31.start
  measures "d76" distance of L31.start L31.end
  measures "d77" distance of L31.start L33.end
extrude "Extrusion20" cut sketch "Skizze20" against normal blind 30 contours L30 L31 L32 L33 L34
sketch "Skizze21" plane through (0, 0, 25) normal (0, 0, 1) x (-1, 0, 0)
  line L0 (-4.516, 12.0187) -> (-6.016, 12.0187)
  line L1 (-6.016, 12.0187) -> (-6.016, 7.5)
  line L2 (-6.016, 7.5) -> (-6.6738, 7.5)
  line L3 (-6.6738, 7.5) -> (-6.6738, 4.0061)
  line L4 (-6.6738, 4.0061) -> (-8.2952, 4.0061)
  arc A0 (-8.7369, 4.0061) -> (-8.2952, 4.0061) centre (-8.516, 8) ccw
  line L5 (-8.7369, 4.0061) -> (-10.4, 4.0061)
  line L6 (-10.4, 4.0061) -> (-10.4, 4.008)
  line L7 (-10.4, 4.008) -> (-11.6, 4.008)
  line L8 (-11.6, 4.008) -> (-11.6, 7.5)
  line L9 (-11.6, 7.5) -> (-12.5254, 7.5)
  line L10 (-12.5254, 7.5) -> (-12.5254, 8)
  line L11 (-12.5254, 8) -> (-12.516, 8)
  line L12 (-12.516, 8) -> (-12.516, 9.5118)
  line L13 (-12.516, 9.5118) -> (-14.216, 9.5118)
  line L14 (-14.216, 9.5118) -> (-14.216, 9.513)
  line L15 (-14.216, 9.513) -> (-14.716, 9.513)
  line L16 (-14.716, 9.513) -> (-14.716, 14.9916)
  line L17 (-14.716, 14.9916) -> (-15.716, 14.9916)
  line L18 (-15.716, 14.9916) -> (-15.716, 17.9916)
  line L19 (-15.716, 17.9916) -> (-14.216, 17.9916)
  line L20 (-14.216, 17.9916) -> (-14.216, 23.0062)
  line L21 (-14.216, 23.0062) -> (-15.716, 23.0062)
  line L22 (-15.716, 23.0062) -> (-15.716, 26.0062)
  line L23 (-15.716, 26.0062) -> (-14.216, 26.0062)
  line L24 (-14.216, 26.0062) -> (-14.216, 30.0118)
  line L25 (-14.216, 30.0118) -> (-12.516, 30.0118)
  line L26 (-12.516, 30.0118) -> (-12.516, 32)
  line L27 (-12.516, 32) -> (-20, 32)
  line L28 (-20, 32) -> (-20, 0)
  line L29 (-20, 0) -> (0, 0)
  line L30 (0, 0) -> (0, 32)
  line L31 (0, 32) -> (-6.016, 32)
  line L32 (-6.016, 32) -> (-6.016, 15.0187)
  line L33 (-6.016, 15.0187) -> (-4.516, 15.0187)
  line L34 (-4.516, 15.0187) -> (-4.516, 12.0187)
  line L35 (-6.016, 11.0245) -> (-4.516, 11.0245)
  line L36 (-4.516, 11.0245) -> (-4.516, 16.0245)
  line L37 (-4.516, 16.0245) -> (-6.016, 16.0245)
  line L38 (-6.016, 16.0245) -> (-6.016, 11.0245)
  dimension "d80" = 5
  constraint horizontal L35
  constraint vertical L36
  constraint horizontal L37
  constraint vertical L38
  constraint coincident L1 L35.start
  measures "d80" distance of L35.start L37.end
extrude "Extrusion21" cut sketch "Skizze21" against normal blind 30 contours L0 L1 L35 L36 L38 | L32 L33 L36 L37 L38
sketch "Skizze22" plane through (0, 0, 25) normal (0, 0, 1) x (-1, 0, 0)
  line L0 (-4.516, 11.0245) -> (-6.016, 11.0245)
  line L1 (-6.016, 11.0245) -> (-6.016, 7.5)
  line L2 (-6.016, 7.5) -> (-6.6738, 7.5)
  line L3 (-6.6738, 7.5) -> (-6.6738, 4.0061)
  line L4 (-6.6738, 4.0061) -> (-8.2952, 4.0061)
  arc A0 (-8.7369, 4.0061) -> (-8.2952, 4.0061) centre (-8.516, 8) ccw
  line L5 (-8.7369, 4.0061) -> (-10.4, 4.0061)
  line L6 (-10.4, 4.0061) -> (-10.4, 4.008)
  line L7 (-10.4, 4.008) -> (-11.6, 4.008)
  line L8 (-11.6, 4.008) -> (-11.6, 7.5)
  line L9 (-11.6, 7.5) -> (-12.5254, 7.5)
  line L10 (-12.5254, 7.5) -> (-12.5254, 8)
  line L11 (-12.5254, 8) -> (-12.516, 8)
  line L12 (-12.516, 8) -> (-12.516, 9.5118)
  line L13 (-12.516, 9.5118) -> (-14.216, 9.5118)
  line L14 (-14.216, 9.5118) -> (-14.216, 9.513)
  line L15 (-14.216, 9.513) -> (-14.716, 9.513)
  line L16 (-14.716, 9.513) -> (-14.716, 14.9916)
  line L17 (-14.716, 14.9916) -> (-15.716, 14.9916)
  line L18 (-15.716, 14.9916) -> (-15.716, 17.9916)
  line L19 (-15.716, 17.9916) -> (-14.216, 17.9916)
  line L20 (-14.216, 17.9916) -> (-14.216, 23.0062)
  line L21 (-14.216, 23.0062) -> (-15.716, 23.0062)
  line L22 (-15.716, 23.0062) -> (-15.716, 26.0062)
  line L23 (-15.716, 26.0062) -> (-14.216, 26.0062)
  line L24 (-14.216, 26.0062) -> (-14.216, 30.0118)
  line L25 (-14.216, 30.0118) -> (-12.516, 30.0118)
  line L26 (-12.516, 30.0118) -> (-12.516, 32)
  line L27 (-12.516, 32) -> (-20, 32)
  line L28 (-20, 32) -> (-20, 0)
  line L29 (-20, 0) -> (0, 0)
  line L30 (0, 0) -> (0, 32)
  line L31 (0, 32) -> (-6.016, 32)
  line L32 (-6.016, 32) -> (-6.016, 16.0245)
  line L33 (-6.016, 16.0245) -> (-4.516, 16.0245)
  line L34 (-4.516, 16.0245) -> (-4.516, 11.0245)
  line L35 (-7.2903, 4.0061) -> (-6.6738, 4.0061)
  line L36 (-6.6738, 4.0061) -> (-6.6738, 7.5)
  line L37 (-6.6738, 7.5) -> (-7.2903, 7.5)
  line L38 (-7.2903, 7.5) -> (-7.2903, 4.0061)
  constraint horizontal L35
  constraint vertical L36
  constraint horizontal L37
  constraint vertical L38
  constraint coincident L2.end L3.start
  constraint coincident L4 L35.start
extrude "Extrusion22" add sketch "Skizze22" against normal blind 25 contours L3 L4 L35 L36 L37 L38
sketch "Skizze23" plane through (0, 0, 25) normal (0, 0, 1) x (-1, 0, 0)
  line L0 (-4.516, 11.0245) -> (-6.016, 11.0245)
  line L1 (-6.016, 11.0245) -> (-6.016, 7.5)
  line L2 (-6.016, 7.5) -> (-7.2903, 7.5)
  line L3 (-7.2903, 7.5) -> (-7.2903, 4.0061)
  line L4 (-7.2903, 4.0061) -> (-8.2952, 4.0061)
  arc A0 (-8.7369, 4.0061) -> (-8.2952, 4.0061) centre (-8.516, 8) ccw
  line L5 (-8.7369, 4.0061) -> (-10.4, 4.0061)
  line L6 (-10.4, 4.0061) -> (-10.4, 4.008)
  line L7 (-10.4, 4.008) -> (-11.6, 4.008)
  line L8 (-11.6, 4.008) -> (-11.6, 7.5)
  line L9 (-11.6, 7.5) -> (-12.5254, 7.5)
  line L10 (-12.5254, 7.5) -> (-12.5254, 8)
  line L11 (-12.5254, 8) -> (-12.516, 8)
  line L12 (-12.516, 8) -> (-12.516, 9.5118)
  line L13 (-12.516, 9.5118) -> (-14.216, 9.5118)
  line L14 (-14.216, 9.5118) -> (-14.216, 9.513)
  line L15 (-14.216, 9.513) -> (-14.716, 9.513)
  line L16 (-14.716, 9.513) -> (-14.716, 14.9916)
  line L17 (-14.716, 14.9916) -> (-15.716, 14.9916)
  line L18 (-15.716, 14.9916) -> (-15.716, 17.9916)
  line L19 (-15.716, 17.9916) -> (-14.216, 17.9916)
  line L20 (-14.216, 17.9916) -> (-14.216, 23.0062)
  line L21 (-14.216, 23.0062) -> (-15.716, 23.0062)
  line L22 (-15.716, 23.0062) -> (-15.716, 26.0062)
  line L23 (-15.716, 26.0062) -> (-14.216, 26.0062)
  line L24 (-14.216, 26.0062) -> (-14.216, 30.0118)
  line L25 (-14.216, 30.0118) -> (-12.516, 30.0118)
  line L26 (-12.516, 30.0118) -> (-12.516, 32)
  line L27 (-12.516, 32) -> (-20, 32)
  line L28 (-20, 32) -> (-20, 0)
  line L29 (-20, 0) -> (0, 0)
  line L30 (0, 0) -> (0, 32)
  line L31 (0, 32) -> (-6.016, 32)
  line L32 (-6.016, 32) -> (-6.016, 16.0245)
  line L33 (-6.016, 16.0245) -> (-4.516, 16.0245)
  line L34 (-4.516, 16.0245) -> (-4.516, 11.0245)
  line L35 (-11.6, 4.008) -> (-7.2957, 4.008)
  line L36 (-7.2957, 4.008) -> (-7.2957, 3.008)
  line L37 (-7.2957, 3.008) -> (-11.6, 3.008)
  line L38 (-11.6, 3.008) -> (-11.6, 4.008)
  dimension "d85" = 1
  constraint horizontal L35
  constraint vertical L36
  constraint horizontal L37
  constraint vertical L38
  constraint coincident L7.end L8.start
  measures "d85" distance of L7.end L37.end
extrude "Extrusion23" cut sketch "Skizze23" against normal blind 25 contours L4 A0 L5 L7 L35 L36 L37 L38
sketch "Skizze24" plane through (0, 0, 0) normal (0, 0, -1) x (1, 0, 0)
  line L0 (11.6, 7.5) -> (11.6, 3.008)
  line L1 (11.6, 3.008) -> (7.2957, 3.008)
  line L2 (7.2957, 3.008) -> (7.2957, 4.0061)
  line L3 (7.2957, 4.0061) -> (7.2903, 4.0061)
  line L4 (7.2903, 4.0061) -> (7.2903, 7.5)
  line L5 (7.2903, 7.5) -> (6.016, 7.5)
  line L6 (6.016, 7.5) -> (6.016, 11.0245)
  line L7 (6.016, 11.0245) -> (4.516, 11.0245)
  line L8 (4.516, 11.0245) -> (4.516, 16.0245)
  line L9 (4.516, 16.0245) -> (6.016, 16.0245)
  line L10 (6.016, 16.0245) -> (6.016, 32)
  line L11 (6.016, 32) -> (0, 32)
  line L12 (0, 32) -> (0, 0)
  line L13 (0, 0) -> (20, 0)
  line L14 (20, 0) -> (20, 32)
  line L15 (20, 32) -> (12.516, 32)
  line L16 (12.516, 32) -> (12.516, 30.0118)
  line L17 (12.516, 30.0118) -> (14.216, 30.0118)
  line L18 (14.216, 30.0118) -> (14.216, 26.0062)
  line L19 (14.216, 26.0062) -> (15.716, 26.0062)
  line L20 (15.716, 26.0062) -> (15.716, 23.0062)
  line L21 (15.716, 23.0062) -> (14.216, 23.0062)
  line L22 (14.216, 23.0062) -> (14.216, 17.9916)
  line L23 (14.216, 17.9916) -> (15.716, 17.9916)
  line L24 (15.716, 17.9916) -> (15.716, 14.9916)
  line L25 (15.716, 14.9916) -> (14.716, 14.9916)
  line L26 (14.716, 14.9916) -> (14.716, 9.513)
  line L27 (14.716, 9.513) -> (14.216, 9.513)
  line L28 (14.216, 9.513) -> (14.216, 9.5118)
  line L29 (14.216, 9.5118) -> (12.516, 9.5118)
  line L30 (12.516, 9.5118) -> (12.516, 8)
  line L31 (12.516, 8) -> (12.5254, 8)
  line L32 (12.5254, 8) -> (12.5254, 7.5)
  line L33 (12.5254, 7.5) -> (11.6, 7.5)
  line L34 (20, 0) -> (0, 0)
  line L35 (0, 0) -> (0, 32)
  line L36 (0, 32) -> (20, 32)
  line L37 (20, 32) -> (20, 0)
  constraint horizontal L34
  constraint vertical L35
  constraint horizontal L36
  constraint vertical L37
  constraint coincident L11.end L12.start
  constraint coincident L13.end L14.start
extrude "Extrusion24" add sketch "Skizze24" along normal blind 5
sketch "Skizze25" plane through (0, 0, 0) normal (-1, 0, 0) x (0, -1, 0)
  line L0 (32, -5) -> (32, 25)
  line L1 (32, 25) -> (0, 25)
  line L2 (0, 25) -> (0, -5)
  line L3 (0, -5) -> (32, -5)
  line L4 (0, -5) -> (0, -9)
  line L5 (0, -9) -> (32, -5)
  constraint coincident L2.end L3.start
  constraint perpendicular L3 L4
  constraint coincident L0.start L3.end
sketch "Skizze30" plane through (20, 0, 0) normal (1, 0, 0) x (0, 1, 0)
  line L0 (0, -5) -> (0, 25)
  line L1 (0, 25) -> (-32, 25)
  line L2 (-32, 25) -> (-32, -5)
  line L3 (-32, -5) -> (0, -5)
sketch "Skizze31" plane through (0, 0, 0) normal (-1, 0, 0) x (0, -1, 0)
  line L0 (32, -5) -> (32, 25)
  line L1 (32, 25) -> (0, 25)
  line L2 (0, 25) -> (0, -5)
  line L3 (0, -5) -> (32, -5)
sketch "Skizze32" plane through (0, 0, 0) normal (-1, 0, 0) x (0, -1, 0)
  line L0 (0, -5) -> (0, -9.5)
  line L1 (0, -9.5) -> (32, -5)
  line L2 (32, -5) -> (0, -5)
  constraint vertical L0
  constraint perpendicular L0 L2
extrude "Extrusion30" add sketch "Skizze32" against normal blind 20
hole "Bohrung5" at (9.4093, -6.812, -8.5421) direction (0, 0.139255, 0.990257) diameter 4.06 depth 11 tip angle 180
sketch "Skizze33" plane through (20, 0, 0) normal (1, 0, 0) x (0, 1, 0)
  line L0 (0, -9.5) -> (0, 25)
  line L1 (0, 25) -> (-32, 25)
  line L2 (-32, 25) -> (-32, -5)
  line L3 (-32, -5) -> (0, -9.5)
  line L4 (0, -5) -> (-32, -5)
  line L5 (-32, -5) -> (0, -9.5)
  line L6 (0, -9.5) -> (0, -5)
  constraint coincident L0 L4.start
  constraint coincident L2.end L3.start
  constraint coincident L0.start L3.end
  constraint parallel L0 L6
extrude "Extrusion31" cut sketch "Skizze33" against normal blind 20 contours L0 L3 L4 L5 L6
sketch "Skizze34" plane through (0, 0, 25) normal (0, 0, 1) x (-1, 0, 0)
  line L0 (-11.6, 3.008) -> (-11.6, 7.5)
  line L1 (-11.6, 7.5) -> (-12.5254, 7.5)
  line L2 (-12.5254, 7.5) -> (-12.5254, 8)
  line L3 (-12.5254, 8) -> (-12.516, 8)
  line L4 (-12.516, 8) -> (-12.516, 9.5118)
  line L5 (-12.516, 9.5118) -> (-14.216, 9.5118)
  line L6 (-14.216, 9.5118) -> (-14.216, 9.513)
  line L7 (-14.216, 9.513) -> (-14.716, 9.513)
  line L8 (-14.716, 9.513) -> (-14.716, 14.9916)
  line L9 (-14.716, 14.9916) -> (-15.716, 14.9916)
  line L10 (-15.716, 14.9916) -> (-15.716, 17.9916)
  line L11 (-15.716, 17.9916) -> (-14.216, 17.9916)
  line L12 (-14.216, 17.9916) -> (-14.216, 23.0062)
  line L13 (-14.216, 23.0062) -> (-15.716, 23.0062)
  line L14 (-15.716, 23.0062) -> (-15.716, 26.0062)
  line L15 (-15.716, 26.0062) -> (-14.216, 26.0062)
  line L16 (-14.216, 26.0062) -> (-14.216, 30.0118)
  line L17 (-14.216, 30.0118) -> (-12.516, 30.0118)
  line L18 (-12.516, 30.0118) -> (-12.516, 32)
  line L19 (-12.516, 32) -> (-20, 32)
  line L20 (-20, 32) -> (-20, 0)
  line L21 (-20, 0) -> (0, 0)
  line L22 (0, 0) -> (0, 32)
  line L23 (0, 32) -> (-6.016, 32)
  line L24 (-6.016, 32) -> (-6.016, 16.0245)
  line L25 (-6.016, 16.0245) -> (-4.516, 16.0245)
  line L26 (-4.516, 16.0245) -> (-4.516, 11.0245)
  line L27 (-4.516, 11.0245) -> (-6.016, 11.0245)
  line L28 (-6.016, 11.0245) -> (-6.016, 7.5)
  line L29 (-6.016, 7.5) -> (-7.2903, 7.5)
  line L30 (-7.2903, 7.5) -> (-7.2903, 4.0061)
  line L31 (-7.2903, 4.0061) -> (-7.2957, 4.0061)
  line L32 (-7.2957, 4.0061) -> (-7.2957, 3.008)
  line L33 (-7.2957, 3.008) -> (-11.6, 3.008)
  line L34 (-12.5, 3) -> (-11.6, 7.5)
  line L35 (-7.2903, 7.5) -> (-6.5, 3)
  line L36 (-6.5, 3) -> (-12.5, 3)
  line L37 (-11.6, 7.5) -> (-7.2903, 7.5)
  constraint coincident L0.end L1.start
  constraint coincident L29.end L30.start
  constraint perpendicular L0 L36
extrude "Extrusion32" cut sketch "Skizze34" against normal blind 25 contours L0 L30 L31 L32 L33 L34 L35 L36 | L0 L30 L31 L32 L33 L37
extrude "Extrusion25" [rolled back] along distance -20 taper angle 0
hole "Bohrung4" [rolled back] hole depth 14 hole diameter 3.95 tip angle 180
sketch "Skizze26" plane through (0, 0, 0) normal (-1, 0, 0) x (0, -1, 0)
  line L0 (32, -5) -> (32, 25)
  line L1 (32, 25) -> (0, 25)
  line L2 (0, 25) -> (0, -9)
  line L3 (0, -9) -> (32, -5)
  line L4 (32, -5) -> (0, -5)
  line L5 (0, -5) -> (0, -9)
  line L6 (32, -5) -> (0, -9)
  constraint coincident L0.start L3.end
  constraint coincident L2 L4.end
  constraint perpendicular L2 L4
  constraint coincident L2.end L3.start
extrude "Extrusion26" [rolled back] along distance -20 taper angle 0
sketch "Skizze27" plane through (0, 0, 0) normal (-1, 0, 0) x (0, -1, 0)
  line L0 (0, -5) -> (32, -5)
  line L1 (32, -5) -> (32, 25)
  line L2 (32, 25) -> (0, 25)
  line L3 (0, 25) -> (0, -5)
  line L4 (0, 25) -> (32, 25)
  line L5 (32, 25) -> (32, 20.0169)
  line L6 (32, 20.0169) -> (0, 20.0169)
  line L7 (0, 20.0169) -> (0, 25)
  constraint horizontal L4
  constraint vertical L5
  constraint horizontal L6
  constraint vertical L7
  constraint coincident L1 L5.end
  constraint coincident L2.end L3.start
extrude "Extrusion27" [rolled back] along distance -20 taper angle 0
sketch "Skizze28" plane through (0, 0, 20.0169) normal (0, 0, 1) x (-1, 0, 0)
  line L0 (-6.016, 32) -> (-6.016, 16.0245)
  line L1 (-6.016, 16.0245) -> (-4.516, 16.0245)
  line L2 (-4.516, 16.0245) -> (-4.516, 11.0245)
  line L3 (-4.516, 11.0245) -> (-6.016, 11.0245)
  line L4 (-6.016, 11.0245) -> (-6.016, 7.5)
  line L5 (-6.016, 7.5) -> (-7.2903, 7.5)
  line L6 (-7.2903, 7.5) -> (-7.2903, 4.0061)
  line L7 (-7.2903, 4.0061) -> (-7.2957, 4.0061)
  line L8 (-7.2957, 4.0061) -> (-7.2957, 3.008)
  line L9 (-7.2957, 3.008) -> (-11.6, 3.008)
  line L10 (-11.6, 3.008) -> (-11.6, 7.5)
  line L11 (-11.6, 7.5) -> (-12.5254, 7.5)
  line L12 (-12.5254, 7.5) -> (-12.5254, 8)
  line L13 (-12.5254, 8) -> (-12.516, 8)
  line L14 (-12.516, 8) -> (-12.516, 9.5118)
  line L15 (-12.516, 9.5118) -> (-14.216, 9.5118)
  line L16 (-14.216, 9.5118) -> (-14.216, 9.513)
  line L17 (-14.216, 9.513) -> (-14.716, 9.513)
  line L18 (-14.716, 9.513) -> (-14.716, 14.9916)
  line L19 (-14.716, 14.9916) -> (-15.716, 14.9916)
  line L20 (-15.716, 14.9916) -> (-15.716, 17.9916)
  line L21 (-15.716, 17.9916) -> (-14.216, 17.9916)
  line L22 (-14.216, 17.9916) -> (-14.216, 23.0062)
  line L23 (-14.216, 23.0062) -> (-15.716, 23.0062)
  line L24 (-15.716, 23.0062) -> (-15.716, 26.0062)
  line L25 (-15.716, 26.0062) -> (-14.216, 26.0062)
  line L26 (-14.216, 26.0062) -> (-14.216, 30.0118)
  line L27 (-14.216, 30.0118) -> (-12.516, 30.0118)
  line L28 (-12.516, 30.0118) -> (-12.516, 32)
  line L29 (-12.516, 32) -> (-20, 32)
  line L30 (-20, 32) -> (-20, 0)
  line L31 (-20, 0) -> (0, 0)
  line L32 (0, 0) -> (0, 32)
  line L33 (0, 32) -> (-6.016, 32)
  line L34 (-7.2903, 7.5) -> (-6.5, 3)
  line L35 (-6.5, 3) -> (-7.2957, 3.008)
  line L36 (-7.2957, 3.008) -> (-7.2903, 7.5)
  line L37 (-11.6, 7.5) -> (-12.4277, 3.008)
  line L38 (-12.4277, 3.008) -> (-11.6, 3.008)
  line L39 (-11.6, 7.5) -> (-11.6, 3.008)
  constraint coincident L5.end L6.start
  constraint coincident L8.end L9.start
  constraint coincident L10.end L11.start
  constraint coincident L9.end L10.start
  constraint perpendicular L10 L38
extrude "Extrusion28" [rolled back] along distance -20 taper angle 0
sketch "Skizze29" plane through (0, 0, 20.0169) normal (0, 0, 1) x (-1, 0, 0)
  line L0 (-7.2903, 7.5) -> (-6.5, 3)
  line L1 (-6.5, 3) -> (-7.2957, 3.008)
  line L2 (-7.2957, 3.008) -> (-12.4277, 3.008)
  line L3 (-12.4277, 3.008) -> (-11.6, 7.5)
  line L4 (-11.6, 7.5) -> (-12.5254, 7.5)
  line L5 (-12.5254, 7.5) -> (-12.5254, 8)
  line L6 (-12.5254, 8) -> (-12.516, 8)
  line L7 (-12.516, 8) -> (-12.516, 9.5118)
  line L8 (-12.516, 9.5118) -> (-14.216, 9.5118)
  line L9 (-14.216, 9.5118) -> (-14.216, 9.513)
  line L10 (-14.216, 9.513) -> (-14.716, 9.513)
  line L11 (-14.716, 9.513) -> (-14.716, 14.9916)
  line L12 (-14.716, 14.9916) -> (-15.716, 14.9916)
  line L13 (-15.716, 14.9916) -> (-15.716, 17.9916)
  line L14 (-15.716, 17.9916) -> (-14.216, 17.9916)
  line L15 (-14.216, 17.9916) -> (-14.216, 23.0062)
  line L16 (-14.216, 23.0062) -> (-15.716, 23.0062)
  line L17 (-15.716, 23.0062) -> (-15.716, 26.0062)
  line L18 (-15.716, 26.0062) -> (-14.216, 26.0062)
  line L19 (-14.216, 26.0062) -> (-14.216, 30.0118)
  line L20 (-14.216, 30.0118) -> (-12.516, 30.0118)
  line L21 (-12.516, 30.0118) -> (-12.516, 32)
  line L22 (-12.516, 32) -> (-20, 32)
  line L23 (-20, 32) -> (-20, 0)
  line L24 (-20, 0) -> (0, 0)
  line L25 (0, 0) -> (0, 32)
  line L26 (0, 32) -> (-6.016, 32)
  line L27 (-6.016, 32) -> (-6.016, 16.0245)
  line L28 (-6.016, 16.0245) -> (-4.516, 16.0245)
  line L29 (-4.516, 16.0245) -> (-4.516, 11.0245)
  line L30 (-4.516, 11.0245) -> (-6.016, 11.0245)
  line L31 (-6.016, 11.0245) -> (-6.016, 7.5)
  line L32 (-6.016, 7.5) -> (-7.2903, 7.5)
  line L33 (-7.0469, 3.0055) -> (-7.6, 3.0055)
  line L34 (-7.6, 3.0055) -> (-7.6, 5.2)
  line L35 (-7.6, 5.2) -> (-7.0469, 5.2)
  line L36 (-7.0469, 5.2) -> (-7.0469, 3.0055)
  constraint horizontal L33
  constraint vertical L34
  constraint horizontal L35
  constraint vertical L36
  constraint coincident L1 L33.start
extrude "Extrusion29" [rolled back] along distance -20 taper angle 0
hole "Bohrung3" [suppressed]
sketch "Skizze11" plane through (0, 0, 25) normal (0, 0, 1) x (-1, 0, 0)
  arc A0 (-12.516, 9.6788) -> (-4.516, 9.4178) centre (-8.5831, 7.492) ccw
  line L0 (-12.516, 9.6788) -> (-12.516, 10.0118)
  line L1 (-12.516, 10.0118) -> (-14.216, 10.0118)
  line L2 (-14.216, 10.0118) -> (-14.216, 15.5114)
  line L3 (-14.216, 15.5114) -> (-14.516, 15.5114)
  line L4 (-14.516, 15.5114) -> (-14.516, 15.5)
  line L5 (-14.516, 15.5) -> (-15.716, 15.5)
  line L6 (-15.716, 15.5) -> (-15.716, 17.5114)
  line L7 (-15.716, 17.5114) -> (-14.216, 17.5114)
  line L8 (-14.216, 17.5114) -> (-14.216, 23.5233)
  line L9 (-14.216, 23.5233) -> (-15.716, 23.5233)
  line L10 (-15.716, 23.5233) -> (-15.716, 25.5)
  line L11 (-15.716, 25.5) -> (-14.516, 25.5)
  line L12 (-14.516, 25.5) -> (-14.516, 25.5233)
  line L13 (-14.516, 25.5233) -> (-14.216, 25.5233)
  line L14 (-14.216, 25.5233) -> (-14.216, 30.0118)
  line L15 (-14.216, 30.0118) -> (-12.516, 30.0118)
  line L16 (-12.516, 30.0118) -> (-12.516, 32)
  line L17 (-12.516, 32) -> (-20, 32)
  line L18 (-20, 32) -> (-20, 0)
  line L19 (-20, 0) -> (0, 0)
  line L20 (0, 0) -> (0, 32)
  line L21 (0, 32) -> (-4.516, 32)
  line L22 (-4.516, 32) -> (-4.516, 9.4178)
  line L23 (-14.216, 15.0301) -> (-15.75, 15.0301)
  line L24 (-15.75, 15.0301) -> (-15.75, 17.9846)
  line L25 (-15.75, 17.9846) -> (-14.216, 17.9846)
  line L26 (-14.216, 17.9846) -> (-14.216, 15.0301)
  line L27 (-14.216, 22.9549) -> (-15.75, 22.9549)
  line L28 (-15.75, 22.9549) -> (-15.75, 26.0198)
  line L29 (-15.75, 26.0198) -> (-14.216, 26.0198)
  line L30 (-14.216, 26.0198) -> (-14.216, 22.9549)
  constraint horizontal L23
  constraint vertical L24
  constraint horizontal L25
  constraint vertical L26
  constraint coincident L2 L23.start
  constraint horizontal L27
  constraint vertical L28
  constraint horizontal L29
  constraint vertical L30
  constraint coincident L8 L27.start
extrude "Extrusion11" [suppressed]
hole "Bohrung2" [suppressed]
sketch "Skizze9" plane through (0, 0, 25) normal (0, 0, 1) x (-1, 0, 0)
  arc A0 (-12.516, 8.2132) -> (-4.516, 8.1214) centre (-8.5397, 6.1064) ccw
  line L0 (-12.516, 8.2132) -> (-12.516, 10.0118)
  line L1 (-12.516, 10.0118) -> (-14.216, 10.0118)
  line L2 (-14.216, 10.0118) -> (-14.216, 15.5114)
  line L3 (-14.216, 15.5114) -> (-14.516, 15.5114)
  line L4 (-14.516, 15.5114) -> (-14.516, 15.5)
  line L5 (-14.516, 15.5) -> (-15.716, 15.5)
  line L6 (-15.716, 15.5) -> (-15.716, 17.5114)
  line L7 (-15.716, 17.5114) -> (-14.216, 17.5114)
  line L8 (-14.216, 17.5114) -> (-14.216, 23.5233)
  line L9 (-14.216, 23.5233) -> (-15.716, 23.5233)
  line L10 (-15.716, 23.5233) -> (-15.716, 25.5)
  line L11 (-15.716, 25.5) -> (-14.516, 25.5)
  line L12 (-14.516, 25.5) -> (-14.516, 25.5233)
  line L13 (-14.516, 25.5233) -> (-14.216, 25.5233)
  line L14 (-14.216, 25.5233) -> (-14.216, 30.0118)
  line L15 (-14.216, 30.0118) -> (-12.516, 30.0118)
  line L16 (-12.516, 30.0118) -> (-12.516, 32)
  line L17 (-12.516, 32) -> (-20, 32)
  line L18 (-20, 32) -> (-20, 0)
  line L19 (-20, 0) -> (0, 0)
  line L20 (0, 0) -> (0, 32)
  line L21 (0, 32) -> (-4.516, 32)
  line L22 (-4.516, 32) -> (-4.516, 8.1214)
  line L23 (-12.516, 10.0118) -> (-14.216, 10.0118)
  line L24 (-14.216, 10.0118) -> (-14.216, 9.5118)
  line L25 (-14.216, 9.5118) -> (-12.516, 9.5118)
  line L26 (-12.516, 9.5118) -> (-12.516, 10.0118)
  dimension "d37" = 0.5
  constraint horizontal L23
  constraint vertical L24
  constraint horizontal L25
  constraint vertical L26
  constraint coincident L0.end L1.start
  measures "d37" distance of L0.end L25.end
extrude "Extrusion9" [suppressed]